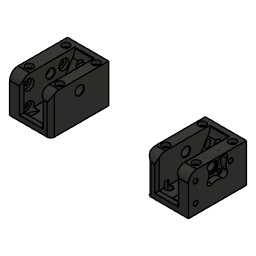
wheel stand mount v15 (Autodesk Fusion 360 design; units mm, degrees)
Autodesk Fusion 360 part; units mm, degrees
sketch "Sketch1" plane through (0, 0, 0) normal (0, 0, 1) x (1, 0, 0)
  line L0 (0, 0) -> (0, 80)
  line L1 (0, 80) -> (25, 80)
  line L2 (25, 80) -> (25, 15)
  line L3 (25, 15) -> (65.2, 15)
  line L4 (65.2, 15) -> (65.2, 80)
  line L5 (65.2, 80) -> (85.2, 80)
  line L6 (0, 0) -> (85.2, 0)
  line L7 (85.2, 0) -> (85.2, 80)
  dimension "d1" = 80
  dimension "d2" = 25
  dimension "d3" = 40.2
  dimension "d4" = 20
  dimension "d5" = 15
  constraint coincident L0.start L6.start
  constraint vertical L0
  constraint perpendicular L0 L1
  constraint perpendicular L1 L2
  constraint perpendicular L2 L3
  constraint perpendicular L3 L4
  constraint perpendicular L4 L5
  constraint perpendicular L0 L6
  constraint perpendicular L5 L7
  constraint collinear L1 L5
  measures "d1" distance of L0.start L0.end
  measures "d2" distance of L0.end L1.end
  measures "d3" distance of L2.end L3.end
  measures "d4" distance of L4.end L5.end
  measures "d5" distance of L3 L6
extrude "Extrude1" add sketch "Sketch1" against normal blind 110 makes body 1
extrude "Extrude9" add 1 faces at (8.3333, 31.6667, 0) along direction (0, 0, 1) blind 10 on bodies 1 bodies 1
sketch "Sketch2" plane through (85.2, 0, 0) normal (1, 0, 0) x (0, 0, -1)
  line L0 (-10, 0) -> (110, 0)
  line L1 (110, 0) -> (110, 80)
  line L2 (110, 80) -> (-10, 80)
  line L3 (50, 80) -> (50, 0) construction
  circle A0 centre (50, 57.5) radius 9.025
  line L4 (-10, 80) -> (-10, 0)
  dimension "d9" = 60
  dimension "d10" = 18.05
  dimension "d119" = 22.5
  constraint coincident L2 L3.start
  constraint coincident L0 L3.end
  constraint perpendicular L0 L3
  constraint coincident L3 A0.centre
  measures "d9" distance of L1 L3
  measures "d10" diameter of A0
  measures "d119" distance of L2 A0.centre
extrude "Extrude2" cut sketch "Sketch2" against normal blind 160 contours A0 bodies 1
sketch "Sketch3" plane through (0, 0, 0) normal (-1, 0, 0) x (0, 0, 1)
  line L0 (10, 80) -> (-110, 80)
  line L1 (-110, 80) -> (-110, 0)
  line L2 (-110, 0) -> (10, 0)
  circle A0 centre (-50, 57.5) radius 12.6
  line L3 (-64.1421, 43.3579) -> (-35.8579, 71.6421) construction
  circle A1 centre (-64.1421, 43.3579) radius 3.25
  circle A2 centre (-35.8579, 71.6421) radius 3.25
  circle A3 centre (-64.1421, 71.6421) radius 3.25
  circle A4 centre (-35.8579, 43.3579) radius 3.25
  circle A5 centre (-64.1421, 43.3579) radius 7
  circle A6 centre (-35.8579, 43.3579) radius 7
  circle A7 centre (-35.8579, 71.6421) radius 7
  circle A8 centre (-64.1421, 71.6421) radius 7
  arc A9 (-70.2713, 46.7391) -> (-70.2713, 68.2609) centre (-89.7775, 57.5) ccw
  line L4 (-64.1421, 71.6421) -> (-35.8579, 43.3579) construction
  arc A10 (-60.7609, 77.7713) -> (-39.2391, 77.7713) centre (-50, 97.2775) ccw
  arc A11 (-29.7287, 68.2609) -> (-29.7287, 46.7391) centre (-10.2225, 57.5) ccw
  arc A12 (-39.2391, 37.2287) -> (-60.7609, 37.2287) centre (-50, 17.7225) ccw
  line L5 (-67.5, 57.5) -> (-32.5, 57.5) construction
  circle A13 centre (-50, 57.5) radius 9.025
  line L6 (10, 0) -> (10, 80)
  dimension "d13" = 25.2
  dimension "d16" = 40
  dimension "d17" = 6.5
  dimension "d19" = 14
  dimension "d25" = 40
  dimension "d26" = 45
  dimension "d27" = 35
  constraint coincident L3.start A1.centre
  constraint coincident L3.end A2.centre
  constraint equal A1 A3
  constraint equal A3 A4
  constraint equal A1 A2
  constraint concentric A1 A5
  constraint concentric A4 A6
  constraint concentric A2 A7
  constraint concentric A3 A8
  constraint equal A5 A8
  constraint equal A7 A8
  constraint equal A6 A7
  constraint tangent A8 A9
  constraint coincident A8 A9.end
  constraint coincident A5 A9.start
  constraint tangent A5 A9
  constraint coincident A3.centre A8.centre
  constraint coincident A4.centre A6.centre
  constraint midpoint A0.centre L4
  constraint perpendicular L3 L4
  constraint symmetric A9.start L4 A10.end
  constraint symmetric A9.end L4 A10.start
  constraint symmetric A9 L4 A10
  constraint symmetric L3 A9.start A12.end
  constraint symmetric L3 A9.end A12.start
  constraint symmetric L3 A9 A12
  constraint symmetric L3 A10.end A11.start
  constraint symmetric L3 A10.start A11.end
  constraint symmetric L3 A10 A11
  constraint midpoint A9 L5.start
  constraint midpoint A11 L5.end
  constraint horizontal L5
  constraint coincident A0.centre A13.centre
  constraint midpoint A0.centre L3
  measures "d13" diameter of A0
  measures "d16" distance of L3.start L3.end
  measures "d17" diameter of A1
  measures "d19" diameter of A5
  measures "d25" distance of A3.centre A4.centre
  measures "d26" angle of L2 L4
  measures "d27" distance of L5.start L5.end
extrude "Extrude3" cut sketch "Sketch3" against normal blind 13 contours A0 | A13 bodies 1
extrude "Extrude4" cut sketch "Sketch3" against normal blind 11 contours A0 | A1 | A2 | A3 | A4 | A5 | A5 A6 A7 A8 A9 A10 A11 A12 | A8 | A6 | A7 | A13 bodies 1
extrude "Extrude5" cut sketch "Sketch3" against normal blind 18 contours A1 | A2 | A3 | A4 bodies 1
sketch "Sketch5" plane through (0, 80, 0) normal (0, 1, 0) x (-1, 0, 0)
  line L0 (-25, 10) -> (-25, -110)
  line L1 (-25, -110) -> (0, -110)
  line L2 (0, -110) -> (0, 10)
  line L3 (-12.5, 10) -> (-12.5, -110) construction
  circle A0 centre (-12.5, -94.025) radius 4.25
  circle A1 centre (-12.5, -18.475) radius 4.25
  line L4 (-13, -59.025) -> (-13, -40.975)
  line L5 (-25, -59.025) -> (-25, -40.975)
  circle A2 centre (-12.5, -94.025) radius 7.5
  circle A3 centre (-12.5, -18.475) radius 7.5
  line L6 (-85.2, 10) -> (-85.2, -110)
  line L7 (-85.2, -110) -> (-65.2, -110)
  line L8 (-65.2, -110) -> (-65.2, 10)
  line L9 (-75.2, 10) -> (-75.2, -110) construction
  line L10 (-12.5, -94.025) -> (-75.2, -94.025) construction
  line L11 (-12.5, -18.475) -> (-75.2, -18.475) construction
  circle A4 centre (-75.2, -18.475) radius 7.5
  circle A5 centre (-75.2, -18.475) radius 4.25
  circle A6 centre (-75.2, -94.025) radius 7.5
  circle A7 centre (-75.2, -94.025) radius 4.25
  line L12 (0, 10) -> (-25, 10)
  line L13 (-65.2, 10) -> (-85.2, 10)
  dimension "d38" = 8.5
  dimension "d39" = 8.5
  dimension "d41" = 22.5
  dimension "d42" = 35
  dimension "d43" = 15
  dimension "d44" = 15
  constraint midpoint L1 L3.end
  constraint coincident L3 A0.centre
  constraint coincident L3 A1.centre
  constraint concentric A0 A2
  constraint concentric A1 A3
  constraint midpoint L7 L9.end
  constraint coincident A0.centre A2.centre
  constraint coincident L9 L10.end
  constraint perpendicular L9 L10
  constraint coincident A1.centre A3.centre
  constraint coincident L9 L11.end
  constraint perpendicular L9 L11
  constraint coincident L11.end A4.centre
  constraint concentric A4 A5
  constraint coincident L10.end A6.centre
  constraint concentric A6 A7
  constraint equal A0 A7
  constraint equal A5 A7
  constraint equal A4 A6
  constraint equal A2 A6
  constraint coincident L3.start L12
  constraint coincident L9.start L13
  constraint midpoint L3.start L12
  constraint midpoint L9.start L13
  measures "d38" diameter of A0
  measures "d39" diameter of A1
  measures "d41" vertical distance of A1.centre L4.end
  measures "d42" vertical distance of A0.centre L4.start
  measures "d43" diameter of A2
  measures "d44" diameter of A3
extrude "Extrude6" cut sketch "Sketch5" against normal blind 140 contours A0 | A1 | A5 | A7 bodies 1
extrude "Extrude7" cut sketch "Sketch5" against normal blind 8 contours A2 | A3 | A4 | A6 bodies 1
sketch "Sketch6" plane through (0, 0, 0) normal (0, -1, 0) x (1, 0, 0)
  circle A0 centre (12.5, -94.025) radius 4.25
  circle A1 centre (12.5, -18.475) radius 4.25
  line L0 (0, 10) -> (0, -110)
  line L1 (0, -110) -> (85.2, -110)
  line L2 (85.2, -110) -> (85.2, 10)
  line L3 (19.05, -14.6934) -> (12.5, -10.9117)
  line L4 (12.5, -10.9117) -> (5.95, -14.6934)
  line L5 (5.95, -14.6934) -> (5.95, -22.2566)
  line L6 (5.95, -22.2566) -> (12.5, -26.0383)
  line L7 (12.5, -26.0383) -> (19.05, -22.2566)
  line L8 (19.05, -22.2566) -> (19.05, -14.6934)
  line L9 (19.05, -90.2434) -> (12.5, -86.4617)
  line L10 (12.5, -86.4617) -> (5.95, -90.2434)
  line L11 (5.95, -90.2434) -> (5.95, -97.8066)
  line L12 (5.95, -97.8066) -> (12.5, -101.5883)
  line L13 (12.5, -101.5883) -> (19.05, -97.8066)
  line L14 (19.05, -97.8066) -> (19.05, -90.2434)
  circle A2 centre (75.2, -18.475) radius 4.25
  circle A3 centre (75.2, -94.025) radius 4.25
  line L15 (68.65, -22.2566) -> (75.2, -26.0383)
  line L16 (75.2, -26.0383) -> (81.75, -22.2566)
  line L17 (81.75, -22.2566) -> (81.75, -14.6934)
  line L18 (81.75, -14.6934) -> (75.2, -10.9117)
  line L19 (75.2, -10.9117) -> (68.65, -14.6934)
  line L20 (68.65, -14.6934) -> (68.65, -22.2566)
  line L21 (68.65, -97.8066) -> (75.2, -101.5883)
  line L22 (75.2, -101.5883) -> (81.75, -97.8066)
  line L23 (81.75, -97.8066) -> (81.75, -90.2434)
  line L24 (81.75, -90.2434) -> (75.2, -86.4617)
  line L25 (75.2, -86.4617) -> (68.65, -90.2434)
  line L26 (68.65, -90.2434) -> (68.65, -97.8066)
  line L27 (85.2, 10) -> (0, 10)
  point P0 (12.5, -18.475)
  point P1 (12.5, -94.025)
  point P2 (75.2, -18.475)
  point P3 (75.2, -94.025)
  dimension "d49" = 13.1
  constraint coincident P0 A1.centre
  constraint coincident A0.centre P1
  constraint vertical L8
  constraint coincident P2 A2.centre
  constraint coincident P3 A3.centre
  constraint equal L8 L20
  constraint equal L20 L26
  constraint vertical L20
  constraint vertical L26
  constraint equal L8 L14
  constraint vertical L14
  measures "d49" distance of L5 L8
extrude "Extrude8" cut sketch "Sketch6" against normal blind 18 contours L3 L4 L5 L6 L7 L8 | L9 L10 L11 L12 L13 L14 | L15 L16 L17 L18 L19 L20 | L21 L22 L23 L24 L25 L26 bodies 1
sketch "Sketch7" plane through (0, 0, -110) normal (0, 0, -1) x (-1, 0, 0)
  line L0 (-85.2, 0) -> (0, 0)
  line L1 (0, 0) -> (0, 80)
  line L2 (0, 80) -> (-25, 80)
  line L3 (-25, 80) -> (-25, 15)
  line L4 (-25, 15) -> (-65.2, 15)
  line L5 (-65.2, 15) -> (-65.2, 80)
  line L6 (-65.2, 80) -> (-85.2, 80)
  line L7 (-85.2, 80) -> (-85.2, 0)
  line L8 (-65.2, 80) -> (-25, 80)
  constraint coincident L5.end L6.start
  constraint coincident L2.end L3.start
extrude "Extrude10" add sketch "Sketch7" against normal blind 10 contours L3 L4 L5 L8 bodies 1
sketch "Sketch8" plane through (25, 0, 0) normal (1, 0, 0) x (0, 0, -1)
  line L0 (100, 15) -> (100, 80)
  line L1 (100, 80) -> (-10, 80)
  line L2 (-10, 80) -> (-10, 15)
  line L3 (-10, 15) -> (100, 15)
  circle A0 centre (50, 57.5) radius 9.025
  line L4 (65, 15) -> (100, 70)
  dimension "d56" = 35
  dimension "d57" = 10
  constraint coincident L3 L4.start
  constraint coincident L0 L4.end
  measures "d56" distance of L0.start L4.start
  measures "d57" distance of L0.end L4.end
extrude "Extrude11" add sketch "Sketch8" along normal blind 43 contours L0 L3 L4 bodies 1
fillet "Fillet1" radius 28 2 edges at (45.1, 15, -65) (45.1, 70, -100) on bodies 1
sketch "Sketch4" plane through (0, 0, 0) normal (-1, 0, 0) x (0, 0, 1)
  arc A0 (-60.7609, 77.7713) -> (-39.2391, 77.7713) centre (-50, 97.2775) ccw
  arc A1 (-29.7287, 68.2609) -> (-39.2391, 77.7713) centre (-35.8579, 71.6421) ccw
  arc A2 (-29.7287, 68.2609) -> (-29.7287, 46.7391) centre (-10.2225, 57.5) ccw
  arc A3 (-39.2391, 37.2287) -> (-29.7287, 46.7391) centre (-35.8579, 43.3579) ccw
  arc A4 (-39.2391, 37.2287) -> (-60.7609, 37.2287) centre (-50, 17.7225) ccw
  arc A5 (-70.2713, 46.7391) -> (-60.7609, 37.2287) centre (-64.1421, 43.3579) ccw
  arc A6 (-70.2713, 46.7391) -> (-70.2713, 68.2609) centre (-89.7775, 57.5) ccw
  arc A7 (-60.7609, 77.7713) -> (-70.2713, 68.2609) centre (-64.1421, 71.6421) ccw
  line L0 (10, 80) -> (-110, 80)
  line L1 (-110, 80) -> (-110, 0)
  line L2 (-110, 0) -> (10, 0)
  line L3 (-5, 80) -> (-5, 0) construction
  line L4 (-77.5, 80) -> (-77.5, 0) construction
  line L5 (-77.5, 60) -> (-5, 60) construction
  line L6 (-5, 20) -> (-77.5, 20) construction
  circle A8 centre (-77.5, 60) radius 10.5
  circle A9 centre (-77.5, 60) radius 4.25
  circle A10 centre (-5, 60) radius 4.25
  circle A11 centre (-5, 20) radius 4.25
  circle A12 centre (-5, 20) radius 10.5
  circle A13 centre (-5, 60) radius 10.5
  circle A14 centre (-77.5, 20) radius 4.25
  circle A15 centre (-77.5, 20) radius 10.5
  line L7 (-77.5, 70) -> (-70.7873, 70) construction
  line L8 (-77.5, 10) -> (-60.7873, 10) construction
  line L9 (10, 0) -> (10, 80)
  dimension "d29" = 20
  dimension "d30" = 20
  dimension "d31" = 21
  dimension "d32" = 8.5
  dimension "d35" = 10
  dimension "d36" = 10
  dimension "d62" = 15
  dimension "d63" = 32.5
  constraint coincident L0 L3.start
  constraint coincident L2 L3.end
  constraint perpendicular L2 L3
  constraint coincident L0 L4.start
  constraint coincident L2 L4.end
  constraint perpendicular L2 L4
  constraint coincident L4 L5.start
  constraint coincident L3 L5.end
  constraint perpendicular L3 L5
  constraint coincident L3 L6.start
  constraint coincident L4 L6.end
  constraint perpendicular L4 L6
  constraint coincident L5.start A8.centre
  constraint concentric A8 A9
  constraint coincident L5.end A10.centre
  constraint coincident L6.start A11.centre
  constraint concentric A11 A12
  constraint concentric A10 A13
  constraint coincident L6.end A14.centre
  constraint concentric A14 A15
  constraint coincident L4 L7.start
  constraint perpendicular L4 L7
  constraint coincident L4 L8.start
  constraint perpendicular L4 L8
  constraint equal A9 A10
  constraint equal A8 A13
  constraint equal A12 A13
  constraint equal A10 A11
  constraint equal A8 A15
  constraint equal A9 A14
  measures "d29" distance of L2 L6
  measures "d30" distance of L0 L5
  measures "d31" diameter of A8
  measures "d32" diameter of A9
  measures "d35" distance of L5 L7
  measures "d36" distance of L6 L8
  measures "d62" distance of L3 L9
  measures "d63" distance of L1 L4
extrude "Extrude12" cut sketch "Sketch4" against normal blind 25 contours A9 | A10 | A11 bodies 1
extrude "Extrude13" cut sketch "Sketch4" along normal blind 6 from surface at -25 contours A6 A8 | A6 A8 | A12 | A13 bodies 1
chamfer "Chamfer1" distance 13.5 distance2 5.5 1 edges at (25, 15, -5) measured on face at (51.8, 15, -17.9542) on bodies 1
sketch "Sketch9" plane through (0, 0, -110) normal (0, 0, -1) x (-1, 0, 0)
  line L0 (-85.2, 0) -> (0, 0)
  line L1 (0, 0) -> (0, 80)
  line L2 (0, 80) -> (-85.2, 80)
  line L3 (-85.2, 80) -> (-85.2, 0)
  line L4 (-65.2, 80) -> (-25, 80)
  line L5 (-42.6, 80) -> (-42.6, 0) construction
  circle A0 centre (-42.6, 20) radius 10.5
  circle A1 centre (-42.6, 60) radius 4.25
  circle A2 centre (-42.6, 20) radius 4.25
  line L6 (-49.1, 56.2472) -> (-42.6, 52.4944)
  line L7 (-42.6, 52.4944) -> (-36.1, 56.2472)
  line L8 (-36.1, 56.2472) -> (-36.1, 63.7528)
  line L9 (-36.1, 63.7528) -> (-42.6, 67.5056)
  line L10 (-42.6, 67.5056) -> (-49.1, 63.7528)
  line L11 (-49.1, 63.7528) -> (-49.1, 56.2472)
  point P0 (-42.6, 60)
  dimension "d79" = 21
  dimension "d80" = 20
  dimension "d81" = 20
  dimension "d82" = 8.5
  dimension "d83" = 8.5
  dimension "d141" = 13
  constraint midpoint L2 L5.start
  constraint perpendicular L2 L5
  constraint coincident L5 A0.centre
  constraint concentric A0 A2
  constraint coincident P0 A1.centre
  constraint coincident L5 P0
  constraint vertical L11
  measures "d79" diameter of A0
  measures "d80" distance of L0 A0.centre
  measures "d81" distance of L2 P0
  measures "d82" diameter of A1
  measures "d83" diameter of A2
  measures "d141" distance of L8 L11
extrude "Extrude16" cut sketch "Sketch9" against normal blind 116 contours A1 | A2 bodies 1
extrude "Extrude17" cut sketch "Sketch9" against normal blind 55.4 from surface at -5 contours A0 | L6 L7 L8 L9 L10 L11 bodies 1
chamfer "Chamfer2" distance 14 distance2 5.4999 1 edges at (42.6, 15, -49.6) measured on face at (56.3, 15, -17.9542) on bodies 1
sketch "Sketch10" plane through (0, 0, 0) normal (0, -1, 0) x (1, 0, 0)
  line L0 (12.5, -86.4617) -> (19.05, -90.2434)
  line L1 (19.05, -90.2434) -> (19.05, -97.8066)
  line L2 (19.05, -97.8066) -> (12.5, -101.5883)
  line L3 (12.5, -101.5883) -> (5.95, -97.8066)
  line L4 (5.95, -97.8066) -> (5.95, -90.2434)
  line L5 (5.95, -90.2434) -> (12.5, -86.4617)
  line L6 (75.2, -101.5883) -> (68.65, -97.8066)
  line L7 (68.65, -97.8066) -> (68.65, -90.2434)
  line L8 (68.65, -90.2434) -> (75.2, -86.4617)
  line L9 (75.2, -86.4617) -> (81.75, -90.2434)
  line L10 (81.75, -90.2434) -> (81.75, -97.8066)
  line L11 (81.75, -97.8066) -> (75.2, -101.5883)
  line L12 (12.5, -10.9117) -> (19.05, -14.6934)
  line L13 (19.05, -14.6934) -> (19.05, -22.2566)
  line L14 (19.05, -22.2566) -> (12.5, -26.0383)
  line L15 (12.5, -26.0383) -> (5.95, -22.2566)
  line L16 (5.95, -22.2566) -> (5.95, -14.6934)
  line L17 (5.95, -14.6934) -> (12.5, -10.9117)
  line L18 (75.2, -26.0383) -> (68.65, -22.2566)
  line L19 (68.65, -22.2566) -> (68.65, -14.6934)
  line L20 (68.65, -14.6934) -> (75.2, -10.9117)
  line L21 (75.2, -10.9117) -> (81.75, -14.6934)
  line L22 (81.75, -14.6934) -> (81.75, -22.2566)
  line L23 (81.75, -22.2566) -> (75.2, -26.0383)
  line L24 (0, 10) -> (0, -110)
  line L25 (0, -110) -> (85.2, -110)
  line L26 (85.2, -110) -> (85.2, 10)
  line L27 (85.2, 10) -> (0, 10)
  circle A0 centre (60, -10) radius 4.25
  circle A1 centre (60, -50) radius 4.25
  line L28 (60, -10) -> (60, -50) construction
  dimension "d93" = 25.2
  dimension "d94" = 20
  dimension "d95" = 40
  dimension "d96" = 8.5
  constraint coincident A0.centre L28.start
  constraint coincident A1.centre L28.end
  constraint vertical L28
  constraint equal A0 A1
  measures "d93" distance of L26 A0.centre
  measures "d94" distance of L27 A0.centre
  measures "d95" vertical distance of A0.centre A1.centre
  measures "d96" diameter of A0
extrude "Extrude18" cut sketch "Sketch10" against normal blind 26 contours A0 | A1 bodies 1
sketch "Sketch11" plane through (0, 15, 0) normal (0, 1, 0) x (-1, 0, 0)
  arc A0 (-55.7662, -49.6295) -> (-64.2338, -49.6295) centre (-60, -50) ccw
  line L0 (-55.7662, -49.6295) -> (-51.8331, -49.6295)
  line L1 (-25, -49.6295) -> (-25, -14.2331)
  line L2 (-25, -14.2331) -> (-38.5, -14.2331)
  line L3 (-38.5, -14.2331) -> (-38.5, 4.2331)
  line L4 (-38.5, 4.2331) -> (-25, 4.2331)
  line L5 (-25, 4.2331) -> (-25, 10)
  line L6 (-25, 10) -> (-65.2, 10)
  line L7 (-65.2, 10) -> (-65.2, -49.6295)
  line L8 (-65.2, -49.6295) -> (-64.2338, -49.6295)
  circle A1 centre (-60, -10) radius 4.25
  line L9 (-53.45, -46.2184) -> (-60, -42.4367)
  line L10 (-60, -42.4367) -> (-66.55, -46.2184)
  line L11 (-66.55, -46.2184) -> (-66.55, -53.7816)
  line L12 (-66.55, -53.7816) -> (-60, -57.5633)
  line L13 (-60, -57.5633) -> (-53.45, -53.7816)
  line L14 (-53.45, -53.7816) -> (-53.45, -46.2184)
  line L15 (-53.45, -6.2184) -> (-60, -2.4367)
  line L16 (-60, -2.4367) -> (-66.55, -6.2184)
  line L17 (-66.55, -6.2184) -> (-66.55, -13.7816)
  line L18 (-66.55, -13.7816) -> (-60, -17.5633)
  line L19 (-60, -17.5633) -> (-53.45, -13.7816)
  line L20 (-53.45, -13.7816) -> (-53.45, -6.2184)
  line L21 (-51.8331, -49.6295) -> (-51.8331, -35.6)
  line L22 (-51.8331, -35.6) -> (-33.3669, -35.6)
  line L23 (-33.3669, -35.6) -> (-33.3669, -49.6295)
  line L24 (-33.3669, -49.6295) -> (-25, -49.6295)
  point P0 (-60, -50)
  point P1 (-60, -10)
  dimension "d99" = 13.1
  constraint coincident P0 A0.centre
  constraint coincident P1 A1.centre
  constraint equal L9 L15
  constraint vertical L14
  constraint vertical L20
  measures "d99" distance of L11 L14
extrude "Extrude19" cut sketch "Sketch11" along normal blind -9 and the other way blind -9 contours A0 L0 L7 L8 L10 L11 L12 L13 L14 | A0 L0 L7 L8 L9 L10 L14 | L7 L16 L17 L18 | L7 L15 L16 L18 L19 L20 | A1 bodies 1
fillet "Fillet3" radius 17.5 2 edges at (12.5, 80, 10) (75.2, 80, 10) on bodies 1
fillet "Fillet3" radius 4.6 3 edges at (45.1, 15, 10) (25, 47.5, 10) (65.2, 47.5, 10) on bodies 1
fillet "Fillet3" radius 7.5 1 edges at (85.2, 40, 10) on bodies 1
chamfer "Chamfer3" distance 0.6 angle 45 4 edges at (79.1624, 72, -20.0119) (79.1624, 72, -95.5619) (16.4624, 72, -95.5619) (16.4624, 72, -20.0119) 7 faces at (6.3333, 19.5768, -0.7711) (6.3333, 59.5768, -0.7711) (12.6667, 59.5768, -73.2711) (38.3711, 59.5768, -108.3333) (38.3711, 19.5768, -108.3333) (64.2289, 2, -10.4232) (64.2289, 2, -50.4232) on bodies 1
chamfer "Chamfer3" distance 1 distance2 0.4 2 faces at (21, 56.6014, -58.9802) (78.5333, 56.6014, -58.9802) on bodies 1
chamfer "Chamfer3" distance 0.4 distance2 0.6 4 edges at (11, 72.8174, -67.1722) (11, 72.8174, -38.8879) (11, 44.5331, -38.8879) (11, 44.5331, -67.1722) measured on face at (11, 42.7088, -43.2308) measured on face at (11, 42.7088, -43.2308) measured on face at (11, 42.7088, -43.2308) measured on face at (11, 42.7088, -43.2308) on bodies 1
sketch "Sketch12" plane through (0, 18, 0) normal (0, -1, 0) x (1, 0, 0)
  circle A0 centre (12.5, -18.475) radius 4.25
  line L0 (19.05, -22.2566) -> (19.05, -15.3078)
  line L1 (19, -14.6645) -> (12.5, -10.9117)
  line L2 (12.5, -10.9117) -> (5.95, -14.6934)
  line L3 (5.95, -14.6934) -> (5.95, -22.2566)
  line L4 (5.95, -22.2566) -> (12.5, -26.0383)
  line L5 (12.5, -26.0383) -> (19.05, -22.2566)
  circle A1 centre (75.2, -18.475) radius 4.25
  line L6 (68.65, -14.6934) -> (68.65, -22.2566)
  line L7 (68.65, -22.2566) -> (75.2, -26.0383)
  line L8 (75.2, -26.0383) -> (81.75, -22.2566)
  line L9 (81.75, -22.2566) -> (81.75, -14.6934)
  line L10 (81.75, -14.6934) -> (75.2, -10.9117)
  line L11 (75.2, -10.9117) -> (68.65, -14.6934)
  circle A2 centre (75.2, -94.025) radius 4.25
  line L12 (68.65, -90.2434) -> (68.65, -97.8066)
  line L13 (68.65, -97.8066) -> (75.2, -101.5883)
  line L14 (75.2, -101.5883) -> (81.75, -97.8066)
  line L15 (81.75, -97.8066) -> (81.75, -90.2434)
  line L16 (81.75, -90.2434) -> (75.2, -86.4617)
  line L17 (75.2, -86.4617) -> (68.65, -90.2434)
  circle A3 centre (12.5, -94.025) radius 4.25
  line L18 (19.05, -97.8066) -> (19.05, -90.2434)
  line L19 (19.05, -90.2434) -> (12.5, -86.4617)
  line L20 (12.5, -86.4617) -> (5.95, -90.2434)
  line L21 (5.95, -90.2434) -> (5.95, -97.8066)
  line L22 (5.95, -97.8066) -> (12.5, -101.5883)
  line L23 (12.5, -101.5883) -> (19.05, -97.8066)
  line L24 (8.25, -88.9155) -> (8.25, -99.1345)
  line L25 (16.75, -88.9155) -> (16.75, -99.1345)
  line L26 (8.25, -89.775) -> (16.75, -89.775)
  line L27 (8.25, -98.275) -> (16.75, -98.275)
  line L28 (19.05, -94.025) -> (68.65, -94.025) construction
  line L29 (43.85, -94.025) -> (43.85, -18.6286) construction
  line L30 (19.05, -18.7822) -> (68.65, -18.475) construction
  line L31 (79.45, -89.775) -> (70.95, -89.775)
  line L32 (70.95, -88.9155) -> (70.95, -99.1345)
  line L33 (79.45, -98.275) -> (70.95, -98.275)
  line L34 (79.45, -88.9155) -> (79.45, -99.1345)
  line L35 (43.85, -56.3268) -> (52, -56.3268) construction
  line L36 (8.25, -22.8786) -> (16.75, -22.8786)
  line L37 (16.75, -23.7382) -> (16.75, -13.5191)
  line L38 (8.25, -14.3786) -> (16.75, -14.3786)
  line L39 (8.25, -23.7382) -> (8.25, -13.5191)
  line L40 (70.95, -23.7382) -> (70.95, -13.5191)
  line L41 (79.45, -22.8786) -> (70.95, -22.8786)
  line L42 (79.45, -23.7382) -> (79.45, -13.5191)
  line L43 (79.45, -14.3786) -> (70.95, -14.3786)
  line L44 (19.05, -15.3078) -> (19, -15.3078)
  line L45 (19, -15.3078) -> (19, -14.6645)
  constraint coincident L20 L24.start
  constraint coincident L22 L24.end
  constraint vertical L24
  constraint coincident L19 L25.start
  constraint coincident L23 L25.end
  constraint parallel L24 L25
  constraint coincident L24 L26.start
  constraint coincident L25 L26.end
  constraint perpendicular L25 L26
  constraint coincident L24 L27.start
  constraint coincident L25 L27.end
  constraint perpendicular L25 L27
  constraint tangent A3 L27
  constraint tangent A3 L26
  constraint tangent A3 L25
  constraint tangent A3 L24
  constraint midpoint L18 L28.start
  constraint midpoint L12 L28.end
  constraint midpoint L28 L29.start
  constraint perpendicular L28 L29
  constraint midpoint L0 L30.start
  constraint midpoint L6 L30.end
  constraint coincident L29.end L30
  constraint symmetric L24.start L29 L34.start
  constraint symmetric L24.end L29 L34.end
  constraint symmetric L25.start L29 L32.start
  constraint symmetric L25.end L29 L32.end
  constraint symmetric L26.start L29 L31.start
  constraint symmetric L26.end L29 L31.end
  constraint symmetric L27.start L29 L33.start
  constraint symmetric L27.end L29 L33.end
  constraint midpoint L29 L35.start
  constraint perpendicular L29 L35
  constraint symmetric L24.start L35 L39.start
  constraint symmetric L24.end L35 L39.end
  constraint symmetric L25.start L35 L37.start
  constraint symmetric L25.end L35 L37.end
  constraint symmetric L26.start L35 L36.start
  constraint symmetric L26.end L35 L36.end
  constraint symmetric L27.start L35 L38.start
  constraint symmetric L27.end L35 L38.end
  constraint symmetric L31.start L35 L41.start
  constraint symmetric L31.end L35 L41.end
  constraint symmetric L32.start L35 L40.start
  constraint symmetric L32.end L35 L40.end
  constraint symmetric L33.start L35 L43.start
  constraint symmetric L33.end L35 L43.end
  constraint symmetric L34.start L35 L42.start
  constraint symmetric L34.end L35 L42.end
extrude "Extrude20" cut sketch "Sketch12" against normal blind 0.2 contours A0 L36 L37 L39 | A0 L0 L1 L2 L3 L4 L5 L37 L38 L39 L44 L45 | A0 L37 L38 | A0 L38 L39 | L4 L5 L36 L37 L39 | A1 L40 L41 L42 | A1 L6 L7 L8 L9 L10 L11 L40 L42 L43 | A1 L42 L43 | A1 L40 L43 | L7 L8 L40 L41 L42 | A2 L33 L34 | A2 L31 L34 | L16 L17 L31 L32 L34 | A2 L31 L32 | A2 L32 L33 | L13 L14 L32 L33 L34 | A3 L25 L27 | A3 L25 L26 | A3 L24 L26 | L19 L20 L24 L25 L26 | A3 L24 L27 | L22 L23 L24 L25 L27 bodies 1
extrude "Extrude21" cut sketch "Sketch12" against normal blind 0.4 contours A0 L36 L37 L39 | A0 L37 L38 | A0 L38 L39 | A1 L40 L41 L42 | A1 L42 L43 | A1 L40 L43 | A2 L33 L34 | A2 L31 L34 | A2 L31 L32 | A2 L32 L33 | A3 L25 L27 | A3 L25 L26 | A3 L24 L26 | A3 L24 L27 bodies 1
chamfer "Chamfer4" distance 1.3 distance2 1.35 2 edges at (65.2, 24, -10) (65.2, 24, -50) measured on face at (65.2, 53.3651, -20.9138) measured on face at (65.2, 53.3651, -20.9138) on bodies 1
sketch "Sketch14" plane through (0, 0, 0) normal (0, -1, 0) x (1, 0, 0)
  circle A0 centre (60, -10) radius 4.85
  arc A1 (85.2, 2.5) -> (77.7, 10) centre (77.7, 2.5) ccw
  line L0 (77.7, 10) -> (0, 10)
  line L1 (0, 10) -> (0, -110)
  line L2 (0, -110) -> (85.2, -110)
  line L3 (85.2, -110) -> (85.2, 2.5)
  line L4 (12.5, -86.4617) -> (19.05, -90.2434)
  line L5 (19.05, -90.2434) -> (19.05, -97.8066)
  line L6 (19.05, -97.8066) -> (12.5, -101.5883)
  line L7 (12.5, -101.5883) -> (5.95, -97.8066)
  line L8 (5.95, -97.8066) -> (5.95, -90.2434)
  line L9 (5.95, -90.2434) -> (12.5, -86.4617)
  line L10 (75.2, -101.5883) -> (68.65, -97.8066)
  line L11 (68.65, -97.8066) -> (68.65, -90.2434)
  line L12 (68.65, -90.2434) -> (75.2, -86.4617)
  line L13 (75.2, -86.4617) -> (81.75, -90.2434)
  line L14 (81.75, -90.2434) -> (81.75, -97.8066)
  line L15 (81.75, -97.8066) -> (75.2, -101.5883)
  line L16 (12.5, -10.9117) -> (19.05, -14.6934)
  line L17 (19.05, -14.6934) -> (19.05, -22.2566)
  line L18 (19.05, -22.2566) -> (12.5, -26.0383)
  line L19 (12.5, -26.0383) -> (5.95, -22.2566)
  line L20 (5.95, -22.2566) -> (5.95, -14.6934)
  line L21 (5.95, -14.6934) -> (12.5, -10.9117)
  line L22 (75.2, -26.0383) -> (68.65, -22.2566)
  line L23 (68.65, -22.2566) -> (68.65, -14.6934)
  line L24 (68.65, -14.6934) -> (75.2, -10.9117)
  line L25 (75.2, -10.9117) -> (81.75, -14.6934)
  line L26 (81.75, -14.6934) -> (81.75, -22.2566)
  line L27 (81.75, -22.2566) -> (75.2, -26.0383)
  circle A2 centre (60, -50) radius 4.85
  circle A3 centre (60, -90) radius 4.2
  line L28 (60, -50) -> (60, -90) construction
  line L29 (66.6, -86.1895) -> (60, -82.379)
  line L30 (60, -82.379) -> (53.4, -86.1895)
  line L31 (53.4, -86.1895) -> (53.4, -93.8105)
  line L32 (53.4, -93.8105) -> (60, -97.621)
  line L33 (60, -97.621) -> (66.6, -93.8105)
  line L34 (66.6, -93.8105) -> (66.6, -86.1895)
  point P0 (60, -90)
  dimension "d130" = 40
  dimension "d131" = 8.4
  dimension "d132" = 13.2
  constraint coincident A2.centre L28.start
  constraint vertical L28
  constraint coincident P0 A3.centre
  constraint vertical L34
  measures "d130" distance of A2.centre P0
  measures "d131" diameter of A3
  measures "d132" distance of L31 L34
extrude "Extrude23" cut sketch "Sketch14" against normal blind 7.4 contours L29 L30 L31 L32 L33 L34 bodies 1
extrude "Extrude24" cut sketch "Sketch14" against normal blind 72 contours A3 bodies 1
sketch "Sketch15" plane through (0, 7.4, 0) normal (0, -1, 0) x (1, 0, 0)
  circle A0 centre (60, -90) radius 4.2
  line L0 (66.6, -93.8105) -> (66.6, -86.1895)
  line L1 (66.6, -86.1895) -> (60, -82.379)
  line L2 (60, -82.379) -> (53.4, -86.1895)
  line L3 (53.4, -86.1895) -> (53.4, -93.8105)
  line L4 (53.4, -93.8105) -> (60, -97.621)
  line L5 (60, -97.621) -> (66.6, -93.8105)
  line L6 (54.0746, -85.8) -> (65.9254, -85.8)
  line L7 (65.9254, -94.2) -> (54.0746, -94.2)
  line L8 (55.8, -85.8) -> (55.8, -94.2)
  line L9 (64.2, -85.8) -> (64.2, -94.2)
  constraint coincident L2 L6.start
  constraint coincident L1 L6.end
  constraint horizontal L6
  constraint coincident L5 L7.start
  constraint coincident L4 L7.end
  constraint perpendicular L0 L7
  constraint tangent A0 L7
  constraint tangent A0 L6
  constraint coincident L6 L8.start
  constraint coincident L7 L8.end
  constraint perpendicular L7 L8
  constraint coincident L6 L9.start
  constraint coincident L7 L9.end
  constraint perpendicular L7 L9
  constraint tangent A0 L8
  constraint tangent A0 L9
extrude "Extrude25" cut sketch "Sketch15" against normal blind 0.4 contours A0 L7 L9 | A0 L6 L9 | A0 L6 L8 | A0 L7 L8 bodies 1
extrude "Extrude26" cut sketch "Sketch15" against normal blind 0.2 contours L0 L1 L5 L6 L7 L9 | L2 L3 L4 L6 L7 L8 bodies 1
ref_plane "WorkPlane1" through (185.2, 40, -50) normal (1, 0, 0) x (0, -1, 0)
mirror "Mirror1" about plane through (185.2, 40, -50) normal (1, 0, 0) of bodies 1 makes body 2
sketch "Sketch13" plane through (0, 0, 0) normal (0, -1, 0) x (1, 0, 0)
  circle A0 centre (60, -10) radius 4.85
  arc A1 (85.2, 2.5) -> (77.7, 10) centre (77.7, 2.5) ccw
  line L0 (77.7, 10) -> (0, 10)
  line L1 (0, 10) -> (0, -110)
  line L2 (0, -110) -> (85.2, -110)
  line L3 (85.2, -110) -> (85.2, 2.5)
  line L4 (12.5, -86.4617) -> (19.05, -90.2434)
  line L5 (19.05, -90.2434) -> (19.05, -97.8066)
  line L6 (19.05, -97.8066) -> (12.5, -101.5883)
  line L7 (12.5, -101.5883) -> (5.95, -97.8066)
  line L8 (5.95, -97.8066) -> (5.95, -90.2434)
  line L9 (5.95, -90.2434) -> (12.5, -86.4617)
  line L10 (75.2, -101.5883) -> (68.65, -97.8066)
  line L11 (68.65, -97.8066) -> (68.65, -90.2434)
  line L12 (68.65, -90.2434) -> (75.2, -86.4617)
  line L13 (75.2, -86.4617) -> (81.75, -90.2434)
  line L14 (81.75, -90.2434) -> (81.75, -97.8066)
  line L15 (81.75, -97.8066) -> (75.2, -101.5883)
  line L16 (12.5, -10.9117) -> (19.05, -14.6934)
  line L17 (19.05, -14.6934) -> (19.05, -22.2566)
  line L18 (19.05, -22.2566) -> (12.5, -26.0383)
  line L19 (12.5, -26.0383) -> (5.95, -22.2566)
  line L20 (5.95, -22.2566) -> (5.95, -14.6934)
  line L21 (5.95, -14.6934) -> (12.5, -10.9117)
  line L22 (75.2, -26.0383) -> (68.65, -22.2566)
  line L23 (68.65, -22.2566) -> (68.65, -14.6934)
  line L24 (68.65, -14.6934) -> (75.2, -10.9117)
  line L25 (75.2, -10.9117) -> (81.75, -14.6934)
  line L26 (81.75, -14.6934) -> (81.75, -22.2566)
  line L27 (81.75, -22.2566) -> (75.2, -26.0383)
  circle A2 centre (60, -50) radius 4.85
  line L28 (76.1917, -26.8838) -> (12.5, -26.0383) construction
  line L29 (12.5, -26.0383) -> (11.5083, -100.7428) construction
  line L30 (11.5083, -100.7428) -> (75.2, -101.5883) construction
  line L31 (75.2, -101.5883) -> (76.1917, -26.8838) construction
  circle A3 centre (310.4, -10) radius 4.85
  arc A4 (292.7, 10) -> (285.2, 2.5) centre (292.7, 2.5) ccw
  line L32 (285.2, 2.5) -> (285.2, -110)
  line L33 (285.2, -110) -> (370.4, -110)
  line L34 (370.4, -110) -> (370.4, 10)
  line L35 (370.4, 10) -> (292.7, 10)
  line L36 (351.35, -90.2434) -> (357.9, -86.4617)
  line L37 (357.9, -86.4617) -> (364.45, -90.2434)
  line L38 (364.45, -90.2434) -> (364.45, -97.8066)
  line L39 (364.45, -97.8066) -> (357.9, -101.5883)
  line L40 (357.9, -101.5883) -> (351.35, -97.8066)
  line L41 (351.35, -97.8066) -> (351.35, -90.2434)
  line L42 (301.75, -97.8066) -> (295.2, -101.5883)
  line L43 (295.2, -101.5883) -> (288.65, -97.8066)
  line L44 (288.65, -97.8066) -> (288.65, -90.2434)
  line L45 (288.65, -90.2434) -> (295.2, -86.4617)
  line L46 (295.2, -86.4617) -> (301.75, -90.2434)
  line L47 (301.75, -90.2434) -> (301.75, -97.8066)
  line L48 (351.35, -14.6934) -> (357.9, -10.9117)
  line L49 (357.9, -10.9117) -> (364.45, -14.6934)
  line L50 (364.45, -14.6934) -> (364.45, -22.2566)
  line L51 (364.45, -22.2566) -> (357.9, -26.0383)
  line L52 (357.9, -26.0383) -> (351.35, -22.2566)
  line L53 (351.35, -22.2566) -> (351.35, -14.6934)
  line L54 (301.75, -22.2566) -> (295.2, -26.0383)
  line L55 (295.2, -26.0383) -> (288.65, -22.2566)
  line L56 (288.65, -22.2566) -> (288.65, -14.6934)
  line L57 (288.65, -14.6934) -> (295.2, -10.9117)
  line L58 (295.2, -10.9117) -> (301.75, -14.6934)
  line L59 (301.75, -14.6934) -> (301.75, -22.2566)
  circle A5 centre (310.4, -50) radius 4.85
  line L60 (357.9, -26.0383) -> (295.0524, -26.1613) construction
  line L61 (295.0524, -26.1613) -> (295.2, -101.5883) construction
  line L62 (295.2, -101.5883) -> (358.0476, -101.4653) construction
  line L63 (358.0476, -101.4653) -> (357.9, -26.0383) construction
  line L64 (60, -82.379) -> (66.6, -86.1895)
  line L65 (66.6, -86.1895) -> (66.6, -93.8105)
  line L66 (66.6, -93.8105) -> (60, -97.621)
  line L67 (60, -97.621) -> (53.4, -93.8105)
  line L68 (53.4, -93.8105) -> (53.4, -86.1895)
  line L69 (53.4, -86.1895) -> (60, -82.379)
  line L70 (303.8, -86.1895) -> (310.4, -82.379)
  line L71 (310.4, -82.379) -> (317, -86.1895)
  line L72 (317, -86.1895) -> (317, -93.8105)
  line L73 (317, -93.8105) -> (310.4, -97.621)
  line L74 (310.4, -97.621) -> (303.8, -93.8105)
  line L75 (303.8, -93.8105) -> (303.8, -86.1895)
  dimension "d123" = 10
  dimension "d124" = 10
  text T0 "LH" font "Arial" height 10 bold align centre middle in box 63.6973 x 74.7111 at (76.1917, -26.8838) x (-0.999912, 0.013274) y (-0.013274, -0.999912) spacing 1 kerned
  text T1 "RH" font "Arial" height 10 bold align centre middle in box 62.8478 x 75.4271 at (357.9, -26.0383) x (-0.999998, -0.001957) y (0.001957, -0.999998) spacing 1 kerned
  constraint coincident L18.end
  constraint coincident L10.start
  constraint coincident L51.end
  constraint coincident L42.end
extrude "Extrude22" cut sketch "Sketch13" against normal blind 1 text T0 T1 bodies 1 2
sketch "Sketch17" plane through (0, 0, 0) normal (-1, 0, 0) x (0, 0, 1)
  circle A0 centre (-5, 60) radius 4.85
  arc A1 (-60.7609, 77.7713) -> (-39.2391, 77.7713) centre (-50, 97.2775) ccw
  arc A2 (-29.7287, 68.2609) -> (-39.2391, 77.7713) centre (-35.8579, 71.6421) ccw
  arc A3 (-29.7287, 68.2609) -> (-29.7287, 46.7391) centre (-10.2225, 57.5) ccw
  arc A4 (-39.2391, 37.2287) -> (-29.7287, 46.7391) centre (-35.8579, 43.3579) ccw
  arc A5 (-39.2391, 37.2287) -> (-60.7609, 37.2287) centre (-50, 17.7225) ccw
  arc A6 (-70.2713, 46.7391) -> (-60.7609, 37.2287) centre (-64.1421, 43.3579) ccw
  arc A7 (-70.2713, 46.7391) -> (-70.2713, 68.2609) centre (-89.7775, 57.5) ccw
  arc A8 (-60.7609, 77.7713) -> (-70.2713, 68.2609) centre (-64.1421, 71.6421) ccw
  arc A9 (10, 62.5) -> (-7.5, 80) centre (-7.5, 62.5) ccw
  line L0 (-7.5, 80) -> (-110, 80)
  line L1 (-110, 80) -> (-110, 0)
  line L2 (-110, 0) -> (10, 0)
  line L3 (10, 0) -> (10, 62.5)
  circle A10 centre (-5, 20) radius 4.85
  circle A11 centre (-77.5, 60) radius 4.85
  line L4 (-50.4, 75) -> (-49.6, 75)
  line L5 (-67.5, 57.5) -> (-32.5, 57.5) construction
  line L6 (-50.4, 75) -> (-50.4, 57.5)
  line L7 (-49.6, 75) -> (-49.6, 57.5)
  line L8 (-50.4, 40) -> (-50.4, 57.5)
  line L9 (-49.6, 40) -> (-49.6, 57.5)
  line L10 (-50.4, 40) -> (-49.6, 40)
  arc A12 (-29.9038, 68.3575) -> (-39.1425, 77.5962) centre (-35.8579, 71.6421) ccw
  arc A13 (-60.8575, 77.5962) -> (-39.1425, 77.5962) centre (-50, 97.2775) ccw
  arc A14 (-60.8575, 77.5962) -> (-70.0962, 68.3575) centre (-64.1421, 71.6421) ccw
  arc A15 (-70.0962, 46.6425) -> (-70.0962, 68.3575) centre (-89.7775, 57.5) ccw
  arc A16 (-70.0962, 46.6425) -> (-60.8575, 37.4038) centre (-64.1421, 43.3579) ccw
  arc A17 (-39.1425, 37.4038) -> (-60.8575, 37.4038) centre (-50, 17.7225) ccw
  arc A18 (-39.1425, 37.4038) -> (-29.9038, 46.6425) centre (-35.8579, 43.3579) ccw
  arc A19 (-29.9038, 68.3575) -> (-29.9038, 46.6425) centre (-10.2225, 57.5) ccw
  line L11 (-54.4, 75.2349) -> (-54.4, 74.8349)
  line L12 (-54.4, 74.8349) -> (-50.4, 72.5255)
  line L13 (-50, 75) -> (-50, 71.4) construction
  line L14 (-45.6, 74.8349) -> (-49.6, 72.5255)
  line L15 (-45.6, 75.2349) -> (-45.6, 74.8349)
  line L16 (-52.4, 40.0715) -> (-52.4, 40.6715)
  line L17 (-52.4, 40.6715) -> (-50.4, 41.8262)
  line L18 (-47.6, 40.0715) -> (-47.6, 40.6715)
  line L19 (-47.6, 40.6715) -> (-49.6, 41.8262)
  dimension "d145" = 0.8
  dimension "d148" = 0.2
  dimension "d149" = 0.4
  dimension "d150" = 4
  dimension "d151" = 30
  dimension "d154" = 30
  dimension "d155" = 2
  dimension "d156" = 0.6
  constraint horizontal L4
  constraint midpoint A1 L4
  constraint midpoint A7 L5.start
  constraint midpoint A3 L5.end
  constraint coincident L5 L6.end
  constraint perpendicular L5 L6
  constraint coincident L5 L7.end
  constraint vertical L7
  constraint symmetric L4.start L5 L8.start
  constraint symmetric L4.end L5 L9.start
  constraint symmetric L5 L6.end L8.end
  constraint symmetric L5 L7.end L9.end
  constraint coincident A13 L11.start
  constraint vertical L11
  constraint coincident L6 L12.end
  constraint midpoint L4 L13.start
  constraint perpendicular L4 L13
  constraint symmetric L11.start L13 L15.start
  constraint symmetric L11.end L13 L14.start
  constraint symmetric L12.end L13 L14.end
  constraint coincident A17 L16.start
  constraint vertical L16
  constraint coincident L8 L17.end
  constraint symmetric L13 L16.start L18.start
  constraint symmetric L13 L16.end L18.end
  constraint symmetric L13 L17.end L19.end
  measures "d145" distance of L4.start L4.end
  measures "d149" distance of L11.start L11.end
  measures "d150" distance of L4.start L11
  measures "d151" angle of L4 L12
  measures "d154" angle of L10 L17
  measures "d155" distance of L8.start L16
  measures "d156" distance of L16.start L16.end
extrude "Extrude28" add sketch "Sketch17" against normal blind 10.5 separate body contours L6 L7 L8 L9 A13 A17 | L6 A13 L11 L12 | L7 A13 L14 L15 | L8 A17 L16 L17 | L9 A17 L18 L19 makes body 3
fillet "Fillet4" radius 1.25 2 edges at (5.25, 72.5255, -50.4) (5.25, 72.5255, -49.6) on bodies 3
copy_body "Body->Comp1" bodies 1 removing the originals makes body 4 in component "wheel stand mount LH"
copy_body "Body->Comp2" bodies 2 removing the originals makes body 5 in component "wheel stand mount RH"
mirror "Mirror2" about plane through (185.2, 40, -50) normal (1, 0, 0) of bodies 3 makes body 6
copy_body "CutPasteBodies1" bodies 6 removing the originals makes body 7 in component "wheel stand mount RH"
copy_body "CutPasteBodies1'" bodies 3 removing the originals makes body 8 in component "wheel stand mount LH"
component "wheel stand mount LH" placed x (1, 0, 0) y (0, 1, 0) z (0, 0, 1) at (0, 0, 0)
component "wheel stand mount RH" placed x (1, 0, 0) y (0, 1, 0) z (0, 0, 1) at (0, 0, 0)
hidden bodies 8 7
equation "d93 = 27 mm - 1.8 mm"
named bodies: "wheel stand mount LH", "wheel stand mount RH"
